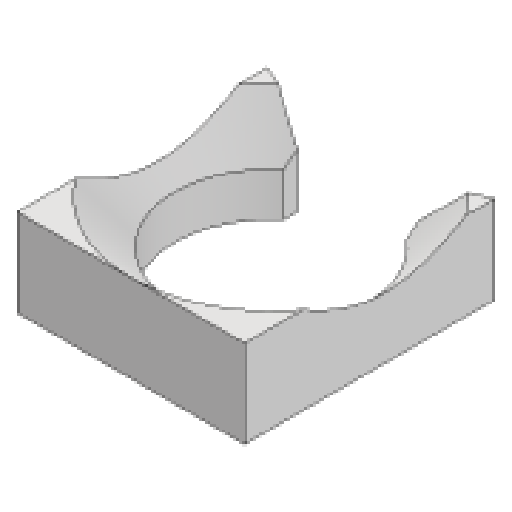
# Autodesk Inventor part: ConeGuide
Saved by Autodesk Inventor 2023 (Build 270158000, 158)
## iProperties
Created: 2022-11-09
Part Number: ConeGuide
Material: Generic
Document SubType Name: Modeling
Designer: deli
Density: 1 g/cm^3
Appearance: Default
Author: deli
Autodesk Inventor part; units mm, degrees
ref_plane "YZ Plane" through (0, 0, 0) normal (1, 0, 0) x (0, 1, 0)
ref_plane "XZ Plane" through (0, 0, 0) normal (0, 1, 0) x (-1, 0, 0)
ref_plane "XY Plane" through (0, 0, 0) normal (0, 0, 1) x (1, 0, 0)
sketch "Sketch1" plane through (0, 0, 0) normal (0, 1, 0) x (-1, 0, 0)
  arc A0 (-188.7669, 580.1191) -> (-245.4654, 580.1191) centre (-217.1161, 627.25) ccw
  circle A1 centre (-217.1161, 627.25) radius 80 construction
  line L0 (-152.1161, 707.25) -> (-282.1161, 707.25)
  line L1 (-282.1161, 707.25) -> (-282.1161, 564.308)
  line L2 (-152.1161, 607.25) -> (-152.1161, 707.25)
  line L3 (-182.1161, 577.25) -> (-182.1161, 627.25)
  line L4 (-252.1161, 577.25) -> (-252.1161, 627.25)
  arc A2 (-182.1161, 627.25) -> (-252.1161, 627.25) centre (-217.1161, 627.25) ccw
  circle A3 centre (-378.1161, 527.25) radius 4
  line L5 (-282.1161, 607.25) -> (-380.5772, 530.4033)
  line L6 (-252.1161, 577.25) -> (-376.5317, 523.5772)
  line L7 (-182.1161, 577.25) -> (-57.7006, 523.5772)
  line L8 (-152.1161, 607.25) -> (-53.6551, 530.4033)
  arc A4 (-57.7006, 523.5772) -> (-53.6551, 530.4033) centre (-56.1161, 527.25) ccw
  line L9 (-152.1161, 607.25) -> (-152.1161, 564.308)
  point P0 (0, 0)
  point P1 (-182.1161, 280.2275)
  point P2 (-115.1514, 290.2976)
  point P3 (-182.1161, 584.8236)
  point P4 (-252.1161, 584.8236)
  dimension "d0" = 110
  dimension "d4" = 10
  dimension "d5" = 10
  dimension "d6" = 70
  dimension "d12" = 8
  dimension "d14" = 100
  dimension "d15" = 50
  dimension "d16" = 100
  dimension "d17" = 100
  dimension "d18" = 160
  dimension "d19" = 100
  constraints: 20 end point, 8 point on circle, 7 tangent, 6 point on line, 5 centre point, 3 equal length, 3 vertical, 1 coincident, 1 concentric, 1 equal radius, 1 horizontal, 1 parallel, 1 perpendicular
  measures "d0" diameter of A0
  measures "d4" distance edge to line of A0 L2
  measures "d5" distance edge to line of A0 L1
  measures "d6" diameter of A2
  measures "d12" diameter of A3
  measures "d15" distance of L4.start L4.end
  measures "d16" vertical distance of A2.centre A3.centre
  measures "d17" distance from line of L0 L5.start
  measures "d18" diameter of A1
  measures "d19" distance from line of L0 L2.start
extrude "Extrusion1" add sketch "Sketch1" along normal blind 50 contours A0 L4 L6 L1 L0 L2 L9 L7 L3
chamfer "Chamfer1" distance 25 angle 45 1 edges at (217.1161, 50, 682.25)
equation "\"d5\" = d4"
equation "\"d19\" = d17"
body "Solid1"
